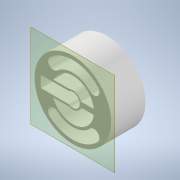
# Autodesk Inventor part: Part5
Saved by Autodesk Inventor 2020 (Build 240168000, 168)
## iProperties
Created: 2022-04-08
Part Number: Part5
Material: Generic
Document SubType Name: Modeling
Designer: Mic
Density: 1 g/cm^3
Appearance: Default
Author: Mic
Autodesk Inventor part; units mm, degrees
ref_plane "YZ Plane" through (0, 0, 0) normal (1, 0, 0) x (0, 1, 0)
ref_plane "XZ Plane" through (0, 0, 0) normal (0, 1, 0) x (-1, 0, 0)
ref_plane "Work Plane1" through (0, 0, -17.4625) normal (0, 0, -1) x (-1, 0, 0)
sketch "Sketch1" plane through (0, 0, -17.4625) normal (0, 0, -1) x (-1, 0, 0)
  line L0 (21.9058, 2.4654) -> (9.8822, 2.4654) projected
  arc A0 (9.8822, 2.4654) -> (9.8822, -2.4654) centre (8.2326, 0) ccw projected
  line L1 (9.8822, -2.4654) -> (21.9058, -2.4654) projected
  arc A1 (21.9058, -2.4654) -> (21.9058, 2.4654) centre (8.2326, 0) ccw projected
  circle A2 centre (8.2326, 0) radius 16.4653 projected
  line L2 (-0.7639, 1.0986) -> (4.7936, 1.0986) projected
  arc A3 (9.6103, 3.3371) -> (4.7936, 1.0986) centre (8.2326, 0) ccw projected
  line L3 (9.6103, 3.3371) -> (16.6593, 3.3371) projected
  arc A4 (16.6593, 3.3371) -> (-0.7639, 1.0986) centre (8.2326, 0) ccw projected
  arc A5 (18.0899, 11.1174) -> (-2.5396, 10.2334) centre (8.2326, 0) ccw projected
  arc A6 (-2.5396, 10.2334) -> (0.8781, 6.9867) centre (-0.8307, 8.61) ccw projected
  arc A7 (14.9625, 7.5902) -> (0.8781, 6.9867) centre (8.2326, 0) ccw projected
  arc A8 (14.9625, 7.5902) -> (18.0899, 11.1174) centre (16.5262, 9.3538) ccw projected
  arc A9 (-2.5396, -10.2334) -> (18.0899, -11.1174) centre (8.2326, 0) ccw projected
  arc A10 (18.0899, -11.1174) -> (14.9625, -7.5902) centre (16.5262, -9.3538) ccw projected
  arc A11 (0.8781, -6.9867) -> (14.9625, -7.5902) centre (8.2326, 0) ccw projected
  arc A12 (0.8781, -6.9867) -> (-2.5396, -10.2334) centre (-0.8307, -8.61) ccw projected
  line L4 (16.6593, -3.3371) -> (9.6103, -3.3371) projected
  arc A13 (4.7936, -1.0986) -> (9.6103, -3.3371) centre (8.2326, 0) ccw projected
  line L5 (4.7936, -1.0986) -> (-0.7639, -1.0986) projected
  arc A14 (-0.7639, -1.0986) -> (16.6593, -3.3371) centre (8.2326, 0) ccw projected
  point P0 (0, 0)
extrude "Extrusion1" add sketch "Sketch1" along normal blind 14.75
ref_plane "Work Plane2" through (-8.2326, 0, -24.8375) normal (0, 0, -1) x (-1, 0, 0)
body "Solid1"
